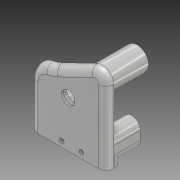
# Autodesk Inventor part: phalanx_3_housing_R
Saved by Autodesk Inventor 2017 SP1 (Build 210196100, 196)
## iProperties
Created: 2017-06-05
Part Number: phalanx_3_housing_R
Material: Generic
Document SubType Name: Modeling
Designer: Tomasz
Density: 1 g/cm^3
Appearance: Aluminum - Polished
shaft_to_encoder_mount_points: 10,700 mm
dist_screw_mount_point_1: 5,250 mm
dist_screw_mount_point_2: 2,250 mm
fingertip_mount_spacing: 15,000 mm
encoder_mount_height: 2,250 mm
fingertip_mounting_dist_from_edge: 2,200 mm
Author: Tomasz
## iProperties of the stored document phalanx_3_housing_R_3DPrint.ipt
Created: 2018-08-20
Part Number: phalanx_3_housing_R_3DPrint
Material: Generic
Document SubType Name: Modeling
Designer: Tomasz
Density: 1 g/cm^3
Appearance: Default
Author: Tomasz
Autodesk Inventor part; units mm, degrees
ref_plane "YZ Plane" through (0, 0, 0) normal (1, 0, 0) x (0, 1, 0)
ref_plane "XZ Plane" through (0, 0, 0) normal (0, 1, 0) x (-1, 0, 0)
ref_plane "XY Plane" through (0, 0, 0) normal (0, 0, 1) x (1, 0, 0)
sketch "Sketch1" plane through (0, 0, 0) normal (0, 1, 0) x (-1, 0, 0)
  line L0 (-5, 4.5) -> (5, 4.5)
  line L1 (10, -0.5) -> (10, -12.2)
  line L2 (10, -12.2) -> (-10, -12.2)
  line L3 (-10, -12.2) -> (-10, -0.5)
  line L4 (0, 0) -> (0, -71.875) construction
  arc A0 (10, -0.5) -> (5, 4.5) centre (5, -0.5) ccw
  arc A1 (-5, 4.5) -> (-10, -0.5) centre (-5, -0.5) ccw
  point P0 (-10, 4.5)
  point P1 (10, 4.5)
  dimension "d0" = 20
  dimension "d1" = 12.2
  dimension "d2" = 4.5
  dimension "d28" = 5
  constraints: 11 end point, 4 point on circle, 4 point on line, 4 tangent, 2 centre point, 2 parallel, 1 equal radius, 1 horizontal, 1 perpendicular, 1 vertical, 1 other
  measures "d0" distance between parallel lines of L3 L1
  measures "d1" distance from line of L2 L4.start
  measures "d2" distance from line of L4.start L0
  measures "d28" radius of A0
extrude "Extrusion1" add sketch "Sketch1" along normal blind 2
sketch "Sketch2" plane through (0, 2, 0) normal (0, 1, 0) x (1, 0, 0)
  circle A0 centre (0, 0) radius 2.5
  dimension "d6" = 5
  constraints: 1 centre point, 1 coincident
  measures "d6" diameter of A0
extrude "Extrusion2" cut sketch "Sketch2" against normal blind 1.5
hole "Hole1" at (0, 0.5, 0) direction (0, -1, 0) diameter 3.5 end through all
sketch "Sketch7" plane through (0, 2, 0) normal (0, 1, 0) x (1, 0, 0)
  line L0 (15, 10.7) -> (-18, 10.7) construction
  line L1 (3.5, 10.7) -> (-1.7, 10.7) construction
  circle A0 centre (0, 0) radius 2.5 projected
  line L2 (-10, 12.2) -> (-10, 0.5) projected
  arc A1 (-10, 0.5) -> (-5, -4.5) centre (-5, 0.5) ccw projected
  line L3 (-5, -4.5) -> (5, -4.5) projected
  arc A2 (5, -4.5) -> (10, 0.5) centre (5, 0.5) ccw projected
  line L4 (10, 0.5) -> (10, 12.2) projected
  line L5 (10, 12.2) -> (-10, 12.2) projected
  line L6 (10, 12.2) -> (-10, 12.2)
  line L7 (-10, 12.2) -> (-10, 9.2)
  line L8 (-10, 9.2) -> (10, 9.2)
  line L9 (10, 9.2) -> (10, 12.2)
  dimension "d44" = 10.7
  dimension "d57" = 3
  constraints: 14 end point, 2 horizontal, 2 parallel, 2 point on line, 1 perpendicular
  measures "d44" distance from line of point (0, 0) L0
  measures "d57" distance between parallel lines of L8 L5
extrude "Extrusion5" add sketch "Sketch7" along normal blind 2.25 contours L5 L4 L8 L2
sketch "Sketch9" plane through (0, 4.25, 0) normal (0, 1, 0) x (1, 0, 0)
  line L0 (-10, 12.2) -> (-10, 9.2) projected
  line L1 (-10, 9.2) -> (10, 9.2) projected
  line L2 (10, 9.2) -> (10, 12.2) projected
  line L3 (10, 12.2) -> (-10, 12.2) projected
  line L4 (0, 0) -> (0, 12.2) construction
  line L5 (-10, 10.7) -> (10, 10.7) construction
  line L6 (10, 0.5) -> (10, 12.2) projected
  point P0 (-1.7, 10.7)
  point P1 (3.5, 10.7)
  dimension "d58" = 3.5
  dimension "d59" = 1.7
  constraints: 4 end point, 3 point on line, 2 midpoint, 1 perpendicular
  measures "d58" distance from line of L4 point (3.5, 10.7)
  measures "d59" distance from line of L4 point (-1.7, 10.7)
hole "Hole5" at (-1.7, 4.25, -10.7) at (3.5, 4.25, -10.7) direction (0, -1, 0) diameter 1.22 end through all
sketch "Sketch10" plane through (0, 0, 0) normal (0, -1, 0) x (1, 0, 0)
  circle A0 centre (-1.7, -10.7) radius 0.61 projected
  circle A1 centre (3.5, -10.7) radius 0.61 projected
  circle A2 centre (0, 0) radius 1.75 projected
  line L0 (-10, -12.2) -> (-10, -0.5) projected
  line L1 (10, -12.2) -> (-10, -12.2) projected
  line L2 (10, -0.5) -> (10, -12.2) projected
  arc A3 (10, -0.5) -> (5, 4.5) centre (5, -0.5) ccw projected
  line L3 (-5, 4.5) -> (5, 4.5) projected
  arc A4 (-5, 4.5) -> (-10, -0.5) centre (-5, -0.5) ccw projected
  line L4 (10, -0.5) -> (10, -9.2) projected
  line L5 (10, -6.95) -> (-10, -6.95) construction
  line L6 (-10, -12.2) -> (-10, -0.5) projected
  line L7 (0, 0) -> (0, -12.2) construction
  arc A5 (10, -6.95) -> (5.5, -6.95) centre (7.75, -6.95) ccw
  arc A6 (-5.5, -6.95) -> (-10, -6.95) centre (-7.75, -6.95) ccw
  line L8 (-10, -9.2) -> (10, -9.2) projected
  line L9 (10, -9.2) -> (-10, -9.2) projected
  arc A7 (5.5, -9.2) -> (10, -9.2) centre (7.75, -9.2) ccw
  line L10 (10, -6.95) -> (10, -9.2)
  line L11 (5.5, -6.95) -> (5.5, -9.2)
  line L12 (-10, -9.2) -> (-10, -6.95)
  line L13 (-5.5, -6.95) -> (-5.5, -9.2)
  circle A8 centre (-7.75, -9.2) radius 2.25
  circle A9 centre (7.75, -9.2) radius 2.25
  dimension "d67" = 5.25
  dimension "d68" = 2.25
  constraints: 13 end point, 12 point on line, 7 point on circle, 3 centre point, 3 coincident, 3 vertical, 2 horizontal alignment, 1 collinear, 1 midpoint, 1 parallel, 1 perpendicular, 1 symmetric about line, 1 vertical alignment, 4 other
  measures "d67" distance between parallel lines of L5 L1
  measures "d68" distance from line of point (7.75, -6.95) L2
sketch "Sketch12" plane through (0, 0, 0) normal (0, -1, 0) x (1, 0, 0)
  circle A0 centre (-1.7, -10.7) radius 0.61 projected
  circle A1 centre (3.5, -10.7) radius 0.61 projected
  circle A2 centre (0, 0) radius 1.75 projected
  line L0 (-10, -12.2) -> (-10, -0.5) projected
  line L1 (10, -12.2) -> (-10, -12.2) projected
  line L2 (10, -0.5) -> (10, -12.2) projected
  arc A3 (10, -0.5) -> (5, 4.5) centre (5, -0.5) ccw projected
  line L3 (-5, 4.5) -> (5, 4.5) projected
  arc A4 (-5, 4.5) -> (-10, -0.5) centre (-5, -0.5) ccw projected
  circle A5 centre (7, 7) radius 3
  line L4 (10, -0.5) -> (10, -12.2) projected
  line L5 (10, -0.5) -> (10, 7)
  arc A6 (10, -0.5) -> (5, 4.5) centre (5, -0.5) ccw projected
  line L6 (-5, 4.5) -> (5.6879, 9.6979)
  line L7 (-5, 4.5) -> (5, 4.5) projected
  dimension "d86" = 7
  dimension "d87" = 7
  constraints: 4 end point, 4 tangent, 2 point on circle, 1 centre point
  measures "d86" horizontal distance of A5.centre point (0, 0)
  measures "d87" horizontal distance of point (0, 0) A5.centre
extrude "Extrusion6" add sketch "Sketch12" against normal up to surface (2 mm away) contours L6 A5 A3 L3 | A3 A5 L5 | A5 A3 | A5 A3
fillet "Fillet2" radius 10 1 edges at (-5, 1, 4.5)
sketch "Sketch13" plane through (0, 2, 0) normal (0, 1, 0) x (1, 0, 0)
  arc A0 (5.6879, -9.6979) -> (10, -7) centre (7, -7) ccw projected
  circle A1 centre (7, -7) radius 3
  point P0 (0, 0)
  constraints: 1 coincident, 1 horizontal alignment, 2 other
extrude "Extrusion7" add sketch "Sketch13" along normal blind 9.15
hole "Hole8" at (7, 11.15, 7) direction (0, -1, 0) diameter 1.5 depth 6.6
sketch "Sketch14" plane through (7, 11.15, 7) normal (0, 1, 0) x (1, 0, 0)
  circle A0 centre (0, 0) radius 0.75 projected
  circle A1 centre (0, 0) radius 3 projected
  circle A2 centre (0, 0) radius 1.25
  point P0 (-7, 7)
  dimension "d102" = 2.5
  constraints: 1 centre point, 1 coincident
  measures "d102" diameter of A2
extrude "Extrusion8" add sketch "Sketch14" along normal blind 0.3 contours A2
extrude "Extrusion9" add sketch "Sketch10" against normal blind 9 contours A8 L8 | L0 A6 L13 A8 | L8 A8 | A9 L11 A5 L2 | A7 L8 | L8 A9
sketch "Sketch11" plane through (10, 0, -12.2) normal (0, 0, -1) x (-1, 0, 0)
  line L0 (10, 0) -> (10, 4.25) construction
  line L1 (0, 0) -> (20, 0) projected
  line L2 (20, 0) -> (20, 4.25) projected
  line L3 (0, 4.25) -> (20, 4.25) projected
  line L4 (0, 0) -> (0, 4.25) projected
  line L5 (0, 0) -> (0, 4.25) projected
  line L6 (0, 2.2) -> (20, 2.2) construction
  point P0 (2.5, 2.2)
  point P1 (17.5, 2.2)
  dimension "d77" = 2.2
  dimension "d78" = 15
  constraints: 4 end point, 4 point on line, 1 midpoint, 1 perpendicular, 1 symmetric about line, 1 vertical
  measures "d77" distance between parallel lines of L6 L1
  measures "d78" distance of point (17.5, 2.2) point (2.5, 2.2)
hole "Hole7" at (7.5, 2.2, -12.2) at (-7.5, 2.2, -12.2) direction (0, 0, 1) diameter 1.6 depth 4
sketch "Sketch15" plane through (0, 9, 0) normal (0, 1, 0) x (1, 0, 0)
  arc A0 (5.5, 6.95) -> (10, 6.95) centre (7.75, 6.95) ccw projected
  arc A1 (-10, 6.95) -> (-5.5, 6.95) centre (-7.75, 6.95) ccw projected
  point P0 (0, 0)
hole "Hole9" at (7.75, 9, -6.95) at (-7.75, 9, -6.95) direction (0, -1, 0) diameter 2 depth 8
fillet "Fillet3" radius 2.1 2 edges at (-5.5, 3.125, -9.2) (5.5, 3.125, -9.2)
fillet "Fillet4" radius 2 9 edges at (8.5912, 0, 9.5432) (1.0936, 0, 7.4635) (-4.7027, 0, 4.7383) (-8.8594, 0, 2.6788) (-10, 0, -3.725) (-10, 0, -10.7) (10, 0, -10.7) (10, 4.25, -10.7) (-10, 4.25, -10.7)
equation "\"d44\" = shaft_to_encoder_mount_points"
equation "\"d48\" = encoder_mount_height"
equation "\"d58\" = encoder_mount_point_1"
equation "\"d59\" = encoder_mount_point_2"
equation "\"d67\" = dist_screw_mount_point_1"
equation "\"d68\" = dist_screw_mount_point_2"
equation "\"d77\" = fingertip_mounting_dist_from_edge"
equation "\"d78\" = fingertip_mount_spacing"
equation "\"shaft_to_encoder_mount_points\" = 10.7"
equation "\"encoder_mount_point_1\" = 3.5"
equation "\"encoder_mount_point_2\" = 1.7"
equation "\"dist_screw_mount_point_1\" = 5.25"
equation "\"dist_screw_mount_point_2\" = 2.25"
equation "\"fingertip_mount_spacing\" = 15"
equation "\"encoder_mount_height\" = 2.25"
equation "\"fingertip_mounting_dist_from_edge\" = 2.2"
body "Solid1"
